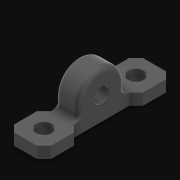
# Autodesk Inventor part: pillowblock
Saved by Autodesk Inventor 2023 (Build 270158000, 158)
## iProperties
Created: 2020-05-27
Part Number: pillowblock
Material: Acetal Resin, Black
Document SubType Name: Modeling
Designer: yuany
Density: 1.09071 g/cm^3
Appearance: Smooth - Black
Author: yuany
Autodesk Inventor part; units mm, degrees
ref_plane "YZ Plane" through (0, 0, 0) normal (1, 0, 0) x (0, 1, 0)
ref_plane "XZ Plane" through (0, 0, 0) normal (0, 1, 0) x (-1, 0, 0)
ref_plane "XY Plane" through (0, 0, 0) normal (0, 0, 1) x (1, 0, 0)
sketch "Sketch1" plane through (0, 0, 0) normal (0, 1, 0) x (-1, 0, 0)
  circle A0 centre (5.08, -5.08) radius 2.1971
  circle A1 centre (5.08, -30.48) radius 2.1971
  line L0 (1.905, 0) -> (8.255, 0)
  line L1 (10.16, -1.905) -> (10.16, -8.255)
  line L2 (8.255, -10.16) -> (1.905, -10.16)
  line L3 (0, -8.255) -> (0, -1.905)
  line L4 (1.905, -25.4) -> (8.255, -25.4)
  line L5 (10.16, -27.305) -> (10.16, -33.655)
  line L6 (8.255, -35.56) -> (1.905, -35.56)
  line L7 (0, -33.655) -> (0, -27.305)
  line L8 (8.255, -10.16) -> (1.905, -10.16)
  line L9 (1.905, -10.16) -> (1.905, -25.4)
  line L10 (1.905, -25.4) -> (8.255, -25.4)
  line L11 (8.255, -25.4) -> (8.255, -10.16)
  line L12 (10.16, -8.255) -> (8.255, -10.16)
  line L13 (8.255, 0) -> (10.16, -1.905)
  line L14 (0, -1.905) -> (1.905, 0)
  line L15 (1.905, -10.16) -> (0, -8.255)
  line L16 (1.905, -25.4) -> (0, -27.305)
  line L17 (1.905, -35.56) -> (0, -33.655)
  line L18 (10.16, -33.655) -> (8.255, -35.56)
  line L19 (8.255, -25.4) -> (10.16, -27.305)
  point P0 (0, 0)
  point P1 (10.16, -10.16)
  point P2 (10.16, 0)
  point P3 (0, -10.16)
  point P4 (0, -25.4)
  point P5 (10.16, -35.56)
  point P6 (10.16, -25.4)
  point P7 (0, -35.56)
  dimension "d2" = 4.3942
  dimension "d3" = 4.3942
  dimension "d4" = 25.4
  dimension "d8" = 10.16
  dimension "d9" = 10.16
  dimension "d10" = 10.16
  dimension "d11" = 10.16
  dimension "d12" = 15.24
  dimension "d13" = 5.08
  dimension "d14" = 5.08
  dimension "d15" = 5.08
  dimension "d16" = 6.35
  dimension "d17" = 1.905
  dimension "d18" = 1.905
  dimension "d19" = 1.905
  dimension "d20" = 1.905
  dimension "d21" = 1.905
  dimension "d22" = 1.905
  dimension "d23" = 1.905
  dimension "d24" = 1.905
  dimension "d25" = 1.905
  dimension "d26" = 1.905
  dimension "d27" = 1.905
  dimension "d28" = 1.905
  dimension "d29" = 1.905
  dimension "d30" = 1.905
  dimension "d31" = 1.905
  dimension "d32" = 1.905
  dimension "d33" = 1.905
  constraints: 40 end point, 18 point on line, 6 parallel, 3 horizontal, 3 perpendicular, 2 centre point, 1 collinear
  measures "d2" diameter of A0
  measures "d3" diameter of A1
  measures "d4" distance of A1.centre A0.centre
  measures "d8" distance of point (10.16, -10.16) point (0, -10.16)
  measures "d9" distance of point (10.16, 0) point (10.16, -10.16)
  measures "d10" distance of point (10.16, -35.56) point (0, -35.56)
  measures "d11" distance of point (10.16, -25.4) point (10.16, -35.56)
  measures "d12" distance between parallel lines of L2 L4
  measures "d13" distance from line of L6 A1.centre
  measures "d14" distance from line of L0 A0.centre
  measures "d15" distance from line of L1 A0.centre
  measures "d16" distance of L10.end L9.end
  measures "d17" distance between parallel lines of L1 L11
  measures "d18" distance of L1.end point (10.16, -10.16)
  measures "d19" distance of L2.start point (10.16, -10.16)
  measures "d20" distance of L0.end point (10.16, 0)
  measures "d21" distance of L1.start point (10.16, 0)
  measures "d22" distance of L3.end point (0, 0)
  measures "d23" distance of L0.start point (0, 0)
  measures "d24" distance of L2.end point (0, -10.16)
  measures "d25" distance of L3.start point (0, -10.16)
  measures "d26" distance of L4.start point (0, -25.4)
  measures "d27" distance of L7.end point (0, -25.4)
  measures "d28" distance of L6.end point (0, -35.56)
  measures "d29" distance of L7.start point (0, -35.56)
  measures "d30" distance of L5.end point (10.16, -35.56)
  measures "d31" distance of L6.start point (10.16, -35.56)
  measures "d32" distance of L4.end point (10.16, -25.4)
  measures "d33" distance of L5.start point (10.16, -25.4)
extrude "Extrusion1" add sketch "Sketch1" along normal blind 3.175
sketch "Sketch2" plane through (0, 0, 0) normal (0, -1, 0) x (1, 0, 0)
  line L0 (-3.3528, -15.5448) -> (-6.8072, -15.5448)
  line L1 (-7.3152, -16.0528) -> (-7.3152, -19.5072)
  line L2 (-6.8072, -20.0152) -> (-3.3528, -20.0152)
  line L3 (-2.8448, -19.5072) -> (-2.8448, -16.0528)
  line L4 (-1.905, -10.16) -> (-1.905, -25.4) projected
  line L5 (-8.255, 0) -> (-1.905, 0) projected
  arc A0 (-2.8448, -16.0528) -> (-3.3528, -15.5448) centre (-3.3528, -16.0528) ccw
  arc A1 (-6.8072, -15.5448) -> (-7.3152, -16.0528) centre (-6.8072, -16.0528) ccw
  arc A2 (-7.3152, -19.5072) -> (-6.8072, -20.0152) centre (-6.8072, -19.5072) ccw
  arc A3 (-3.3528, -20.0152) -> (-2.8448, -19.5072) centre (-3.3528, -19.5072) ccw
  point P0 (0, 0)
  point P1 (-7.3152, -20.0152)
  point P2 (-7.3152, -15.5448)
  point P3 (-2.8448, -20.0152)
  dimension "d36" = 4.4704
  dimension "d37" = 4.4704
  dimension "d38" = 0.9398
  dimension "d39" = 15.5448
  dimension "d40" = 0.508
  constraints: 8 end point, 8 point on circle, 8 tangent, 6 point on line, 4 centre point, 3 equal radius, 2 parallel, 1 horizontal, 1 perpendicular
  measures "d36" distance of point (-2.845, -20.015) point (-7.315, -20.015)
  measures "d37" distance of point (-7.315, -20.015) point (-7.315, -15.545)
  measures "d38" distance between parallel lines of L4 L3
  measures "d39" distance between parallel lines of L5 L0
  measures "d40" radius of A0
extrude "Extrusion2" add sketch "Sketch2" along normal blind 0.6858
sketch "Sketch3" plane through (-1.905, 0, -10.16) normal (1, 0, 0) x (0, 0, -1)
  circle A0 centre (7.62, 6.35) radius 2.1209
  line L0 (0, 0) -> (15.24, 0) projected
  line L1 (7.62, 12.7) -> (7.62, 12.7)
  line L2 (13.97, 6.35) -> (13.97, 0)
  line L3 (13.97, 0) -> (1.27, 0)
  line L4 (1.27, 0) -> (1.27, 6.35)
  arc A1 (7.62, 12.7) -> (1.27, 6.35) centre (7.62, 6.35) ccw
  arc A2 (13.97, 6.35) -> (7.62, 12.7) centre (7.62, 6.35) ccw
  point P0 (-10.16, 0)
  point P1 (13.97, 12.7)
  point P2 (7.62, 12.7)
  point P3 (1.27, 0)
  point P4 (13.97, 0)
  dimension "d43" = 4.2418
  dimension "d44" = 6.35
  dimension "d45" = 7.62
  dimension "d46" = 12.7
  dimension "d47" = 12.7
  dimension "d48" = 6.35
  dimension "d49" = 6.35
  constraints: 8 end point, 4 point on circle, 4 tangent, 3 centre point, 2 parallel, 2 point on line, 1 collinear, 1 concentric, 1 horizontal, 1 perpendicular
  measures "d43" diameter of A0
  measures "d44" distance from line of A0.centre L0
  measures "d45" horizontal distance of A0.centre L0.start
  measures "d46" distance of L2.end L3.end
  measures "d47" distance of point (13.97, 12.7) L2.end
  measures "d48" distance from line of L2 A0.centre
  measures "d49" radius of A1
extrude "Extrusion3" add sketch "Sketch3" against normal up to surface (6.35 mm away)
fillet "Fillet1" radius 1.27 8 edges at (-1.905, 4.7625, -11.43) (-1.905, 4.7625, -24.13) (-1.905, 12.7, -17.78) (-8.255, 4.7625, -11.43) (-8.255, 4.7625, -24.13) (-8.255, 12.7, -17.78) (-5.08, 3.175, -24.13) (-5.08, 3.175, -11.43)
equation "\"d19\" = d18"
equation "\"d20\" = d18"
equation "\"d21\" = d20"
equation "\"d22\" = d18"
equation "\"d23\" = d22"
equation "\"d24\" = d18"
equation "\"d25\" = d24"
equation "\"d26\" = d18"
equation "\"d27\" = d26"
equation "\"d28\" = d18"
equation "\"d29\" = d28"
equation "\"d30\" = d18"
equation "\"d31\" = d30"
equation "\"d32\" = d18"
equation "\"d33\" = d32"
body "Solid1"
